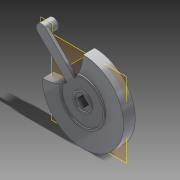
# Autodesk Inventor part: Geneva Drive
Saved by Autodesk Inventor 2018 (Build 220112000, 112)
## iProperties
Created: 2018-01-19
Part Number: Geneva Drive
Material: ABS Plastic
Document SubType Name: Sheet Metal
Designer: Rus
Density: 1.06 g/cm^3
Appearance: Smooth - White
Mass: 73.9959 g
Surface Area: 171.936 cm^2
Volume: 69.8074 cm^3
Sheet Metal Rule: Default
Author: Rus
Autodesk Inventor part; units mm, degrees
ref_plane "YZ Plane" through (0, 0, 0) normal (1, 0, 0) x (0, 1, 0)
ref_plane "XZ Plane" through (0, 0, 0) normal (0, 1, 0) x (-1, 0, 0)
ref_plane "XY Plane" through (0, 0, 0) normal (0, 0, 1) x (1, 0, 0)
sketch "Sketch1" plane through (0, 0, 0) normal (0, 0, 1) x (1, 0, 0)
  line L0 (0, 0) -> (-89.8017, 0) construction
  line L1 (-89.8017, 0) -> (-44.90085, 44.901711) construction
  line L2 (-44.90085, 44.901711) -> (0, 0) construction
  arc A0 (-44.196, 0) -> (0.000848, 44.196) centre (0, 0) ccw
  line L3 (-44.196, 0) -> (-44.196, 44.196848) construction
  line L4 (-44.196, 44.196848) -> (-44.90085, 44.901711) construction
  circle A1 centre (-44.90085, 44.901711) radius 5.715
  arc A2 (-44.196, 0) -> (0.000848, 44.196) centre (-44.196, 44.196848) ccw
  dimension "d8" = 89.8017
  dimension "d9" = 63.5
  dimension "d10" = 63.5
  dimension "d11" = 44.196
  dimension "d12" = 11.43
  constraints: 10 end point, 4 coincident, 4 point on circle, 3 centre point, 1 collinear, 1 horizontal, 1 point on line, 1 vertical
  measures "d8" distance of L0.start L0.end
  measures "d9" distance of L1.end L0.start
  measures "d10" distance of L0.end L1.end
  measures "d11" radius of A0
  measures "d12" diameter of A1
extrude "Extrusion1" add sketch "Sketch1" along normal blind 13.97 and the other way blind 1.27
sketch "Sketch5" plane through (0, 0, 13.97) normal (0, 0, 1) x (1, 0, 0)
  line L0 (2.846729, 10.62373) -> (7.777055, -7.777205)
  line L1 (7.777055, -7.777205) -> (-10.623784, -2.846525)
  line L2 (-10.623784, -2.846525) -> (2.846729, 10.62373)
  line L3 (0, 0) -> (-12.944409, 12.944657) construction
  arc A0 (-44.196, 0) -> (0.000848, 44.196) centre (-44.196, 44.196848) ccw
  dimension "d31" = 19.05
  constraints: 8 end point, 1 coincident, 1 line through centre, 1 perpendicular, 1 point on circle, 7 other
  measures "d31" distance of L1.end L0.start
extrude "Extrusion4" cut sketch "Sketch5" against normal through all
sketch "Sketch6" plane through (0, 0, -1.27) normal (0, 0, -1) x (-1, 0, 0)
  circle A0 centre (0, 0) radius 6.35
  dimension "d34" = 12.7
  constraints: 1 centre point, 1 coincident
  measures "d34" diameter of A0
extrude "Extrusion5" add sketch "Sketch6" along normal blind 8.466667 and the other way blind 21.166667
sketch "Sketch7" plane through (0, 0, 13.97) normal (0, 0, 1) x (1, 0, 0)
  circle A0 centre (0, 0) radius 12.7
  dimension "d39" = 25.4
  constraints: 1 centre point, 1 coincident
  measures "d39" diameter of A0
extrude "Extrusion6" add sketch "Sketch7" against normal up to surface (15.24 mm away)
sketch "Sketch8" plane through (0, 0, -9.736667) normal (0, 0, -1) x (-1, 0, 0)
  circle A0 centre (0, 0) radius 6.35
  line L0 (4.490085, 4.490171) -> (1.64356, -6.133613)
  line L1 (1.64356, -6.133613) -> (-6.133645, 1.643442)
  line L2 (-6.133645, 1.643442) -> (4.490085, 4.490171)
  circle A1 centre (44.90085, 44.901711) radius 5.715
  line L3 (44.90085, 44.901711) -> (0, 0)
  constraints: 8 end point, 1 coincident, 1 point on line, 9 other
extrude "Extrusion7" add sketch "Sketch8" along normal blind 12.7 contours L0 L1 L2
ref_plane "Work Plane1" through (-44.90085, 44.901711, 7.196667) normal (0, 0, -1) x (-1, 0, 0)
sketch "Sketch9" plane through (0, 0, 19.896667) normal (0, 0, 1) x (1, 0, 0)
  circle A0 centre (0, 0) radius 6.35 projected
extrude "Extrusion8" add sketch "Sketch9" along normal blind 1.27
sketch "Sketch10" plane through (0, 0, 13.97) normal (0, 0, 1) x (1, 0, 0)
  circle A0 centre (0, 0) radius 6.35 projected
extrude "Extrusion9" add sketch "Sketch10" along normal blind 8.466667
sketch "Sketch11" plane through (0, 0, 13.97) normal (0, 0, 1) x (1, 0, 0)
  circle A0 centre (0, 0) radius 8.466667
  circle A1 centre (0, 0) radius 10.16
  arc A2 (-44.196, 0) -> (0.000848, 44.196) centre (-44.196, 44.196848) ccw
  arc A3 (-22.076558, 5.933398) -> (-5.932974, 22.076671) centre (0, 0) ccw
  arc A4 (-24.069883, 4.848395) -> (-4.847933, 24.069976) centre (0, 0) ccw
  arc A5 (-44.196, 0) -> (0.000848, 44.196) centre (0, 0) ccw
  circle A6 centre (0, 0) radius 50.8
  point P0 (-37.249283, 0.549345)
  point P1 (-0.548631, 37.249293)
  point P2 (-38.945409, 0.312994)
  point P3 (-0.312247, 38.945415)
  dimension "d51" = 16.93333
  dimension "d52" = 1.69333
  dimension "d53" = 1.69333
  dimension "d55" = 12.7
  dimension "d61" = 101.6
  constraints: 5 centre point, 5 coincident, 4 point on circle, 9 other
  measures "d51" diameter of A0
  measures "d52" radial gap between concentric circles of A1 A0
  measures "d53" radial gap between concentric circles of A4 A3
  measures "d55" radial gap between concentric circles of A3 A1
  measures "d61" diameter of A6
sketch "Sketch11 outline for Extrusion10" plane through (0, 0, 13.97) normal (0, 0, 1) x (1, 0, 0)
  circle A0 centre (0, 0) radius 50.8
  circle A1 centre (0, 0) radius 10.16
  arc A2 (-5.932974, 22.076671) -> (-22.076558, 5.933398) centre (0, 0) cw
  arc A3 (-22.076558, 5.933398) -> (-24.069883, 4.848395) centre (-44.196, 44.196848) cw
  arc A4 (-24.069883, 4.848395) -> (-4.847933, 24.069976) centre (0, 0) ccw
  arc A5 (-4.847933, 24.069976) -> (-5.932974, 22.076671) centre (-44.196, 44.196848) cw
  circle A6 centre (0, 0) radius 8.466667
extrude "Extrusion10" cut sketch "Sketch11 outline for Extrusion10" against normal blind 1.27 draft -10
sketch "Sketch12" plane through (0, 0, 22.436667) normal (0, 0, 1) x (1, 0, 0)
  circle A0 centre (0, 0) radius 6.35 projected
extrude "Extrusion11" add sketch "Sketch12" against normal up to surface (9.736667 mm away)
ref_plane "Work Plane2" through (0, 0, 6.35) normal (0, 0, 1) x (1, 0, 0)
mirror "Mirror1" about plane through (0, 0, 6.35) normal (0, 0, 1) of "Extrusion10"
sketch "Sketch14" plane through (-44.90085, 44.901711, -1.27) normal (0, 0, -1) x (-1, 0, 0)
  circle A0 centre (0, 0) radius 5.715 projected
  point P0 (-44.90085, -44.901711)
extrude "Extrusion12" cut sketch "Sketch14" against normal blind 1.27
sketch "Sketch15" plane through (-44.90085, 44.901711, 13.97) normal (0, 0, 1) x (1, 0, 0)
  circle A0 centre (0, 0) radius 5.715 projected
  point P0 (44.90085, -44.901711)
extrude "Extrusion13" cut sketch "Sketch15" against normal blind 1.27
ref_plane "Work Plane3" through (-12.944409, 12.944657, 0) normal (-0.7071136, -0.7071, 0) x (0.7071, -0.7071136, 0)
sketch "Sketch17" plane through (-12.944409, 12.944657, 0) normal (-0.7071136, -0.7071, 0) x (0.7071, -0.7071136, 0)
  line L0 (-50.908666, 12.7) -> (-39.478666, 12.7)
  line L1 (-39.478666, 12.7) -> (0, 12.7)
  line L2 (0, 12.7) -> (0, 9.313333)
  line L3 (0, 9.313333) -> (-39.478666, 9.313333)
  line L4 (-39.478666, 9.313333) -> (-39.478666, 12.7)
  line L5 (0, 12.7) -> (0, 0)
  line L6 (-39.478666, 12.7) -> (-45.193666, 12.7)
  line L7 (-45.193666, 12.7) -> (-45.193666, 9.313333)
  line L8 (-45.193666, 9.313333) -> (-39.478666, 9.313333)
  line L9 (-39.478666, 9.313333) -> (-39.478666, 12.7)
  line L10 (-39.478666, 0) -> (-50.908666, 0)
  point P0 (18.306334, 0)
  point P1 (-45.193666, 0)
  dimension "d69" = 3.38667
  constraints: 16 end point, 4 parallel, 3 point on line, 2 horizontal, 2 perpendicular, 1 midpoint
  measures "d69" distance between parallel lines of L3 L1
extrude "Extrusion14" add sketch "Sketch17" along normal mid plane 11.43
sketch "Sketch18" plane through (0, 0, -22.436667) normal (0, 0, -1) x (-1, 0, 0)
  circle A0 centre (0, 0) radius 6.35
  dimension "d72" = 12.7
  constraints: 1 centre point, 1 coincident
  measures "d72" diameter of A0
extrude "Extrusion15" cut sketch "Sketch18" against normal through all
sketch "Sketch19" plane through (0, 0, 0) normal (0, 0, -1) x (-1, 0, 0)
  circle A0 centre (0, 0) radius 6.35
  line L0 (6.35, 0.000061) -> (0.000061, -6.35)
  line L1 (0.000061, -6.35) -> (-6.35, -0.000061)
  line L2 (-6.35, -0.000061) -> (-0.000061, 6.35)
  line L3 (-0.000061, 6.35) -> (6.35, 0.000061)
  circle A1 centre (44.90085, 44.901711) radius 5.715 construction
  line L4 (44.90085, 44.901711) -> (0, 0) construction
  constraints: 10 end point, 1 coincident, 1 perpendicular, 11 other
extrude "Extrusion16" add sketch "Sketch19" against normal up to surface (12.7 mm away) contours L3 A0 | A0 L0 | L2 A0 | A0 L1
body "Solid1"
